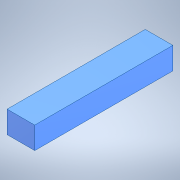
# Autodesk Inventor part: Contenedor Sólido
Saved by Autodesk Inventor 2020.3 (Build 243373000, 373)
## iProperties
Created: 2020-07-19
Part Number: Contenedor Sólido
Material: ABS Plastic
Document SubType Name: Modeling
Designer: juanp
Density: 1.06 g/cm^3
Appearance: Smooth - White
Author: juanp
Autodesk Inventor part; units mm, degrees
ref_plane "YZ Plane" through (0, 0, 0) normal (1, 0, 0) x (0, 1, 0)
ref_plane "XZ Plane" through (0, 0, 0) normal (0, 1, 0) x (-1, 0, 0)
ref_plane "XY Plane" through (0, 0, 0) normal (0, 0, 1) x (1, 0, 0)
sketch "Sketch1" plane through (0, 0, 0) normal (0, 1, 0) x (-1, 0, 0)
  line L0 (0, 0) -> (80, 0)
  line L1 (80, 0) -> (80, -400)
  line L2 (80, -400) -> (0, -400)
  line L3 (0, -400) -> (0, 0)
  line L4 (76, -4) -> (42, -4)
  line L5 (42, -4) -> (42, -39.6)
  line L6 (42, -39.6) -> (76, -39.6)
  line L7 (76, -39.6) -> (76, -4)
  line L8 (76, -43.6) -> (42, -43.6)
  line L9 (42, -43.6) -> (42, -79.2)
  line L10 (42, -79.2) -> (76, -79.2)
  line L11 (76, -79.2) -> (76, -43.6)
  line L12 (76, -83.2) -> (42, -83.2)
  line L13 (42, -83.2) -> (42, -118.8)
  line L14 (42, -118.8) -> (76, -118.8)
  line L15 (76, -118.8) -> (76, -83.2)
  line L16 (76, -122.8) -> (42, -122.8)
  line L17 (42, -122.8) -> (42, -158.4)
  line L18 (42, -158.4) -> (76, -158.4)
  line L19 (76, -158.4) -> (76, -122.8)
  line L20 (76, -162.4) -> (42, -162.4)
  line L21 (42, -162.4) -> (42, -198)
  line L22 (42, -198) -> (76, -198)
  line L23 (76, -198) -> (76, -162.4)
  line L24 (76, -202) -> (42, -202)
  line L25 (42, -202) -> (42, -237.6)
  line L26 (42, -237.6) -> (76, -237.6)
  line L27 (76, -237.6) -> (76, -202)
  line L28 (76, -241.6) -> (42, -241.6)
  line L29 (42, -241.6) -> (42, -277.2)
  line L30 (42, -277.2) -> (76, -277.2)
  line L31 (76, -277.2) -> (76, -241.6)
  line L32 (76, -281.2) -> (42, -281.2)
  line L33 (42, -281.2) -> (42, -316.8)
  line L34 (42, -316.8) -> (76, -316.8)
  line L35 (76, -316.8) -> (76, -281.2)
  line L36 (76, -320.8) -> (42, -320.8)
  line L37 (42, -320.8) -> (42, -356.4)
  line L38 (42, -356.4) -> (76, -356.4)
  line L39 (76, -356.4) -> (76, -320.8)
  line L40 (38, -4) -> (4, -4)
  line L41 (4, -4) -> (4, -39.6)
  line L42 (4, -39.6) -> (38, -39.6)
  line L43 (38, -39.6) -> (38, -4)
  line L44 (38, -43.6) -> (4, -43.6)
  line L45 (4, -43.6) -> (4, -79.2)
  line L46 (4, -79.2) -> (38, -79.2)
  line L47 (38, -79.2) -> (38, -43.6)
  line L48 (38, -83.2) -> (4, -83.2)
  line L49 (4, -83.2) -> (4, -118.8)
  line L50 (4, -118.8) -> (38, -118.8)
  line L51 (38, -118.8) -> (38, -83.2)
  line L52 (38, -122.8) -> (4, -122.8)
  line L53 (4, -122.8) -> (4, -158.4)
  line L54 (4, -158.4) -> (38, -158.4)
  line L55 (38, -158.4) -> (38, -122.8)
  line L56 (38, -162.4) -> (4, -162.4)
  line L57 (4, -162.4) -> (4, -198)
  line L58 (4, -198) -> (38, -198)
  line L59 (38, -198) -> (38, -162.4)
  line L60 (38, -202) -> (4, -202)
  line L61 (4, -202) -> (4, -237.6)
  line L62 (4, -237.6) -> (38, -237.6)
  line L63 (38, -237.6) -> (38, -202)
  line L64 (38, -241.6) -> (4, -241.6)
  line L65 (4, -241.6) -> (4, -277.2)
  line L66 (4, -277.2) -> (38, -277.2)
  line L67 (38, -277.2) -> (38, -241.6)
  line L68 (38, -281.2) -> (4, -281.2)
  line L69 (4, -281.2) -> (4, -316.8)
  line L70 (4, -316.8) -> (38, -316.8)
  line L71 (38, -316.8) -> (38, -281.2)
  line L72 (38, -320.8) -> (4, -320.8)
  line L73 (4, -320.8) -> (4, -356.4)
  line L74 (4, -356.4) -> (38, -356.4)
  line L75 (38, -356.4) -> (38, -320.8)
  line L76 (76, -360.4) -> (4, -360.4)
  line L77 (4, -360.4) -> (4, -396)
  line L78 (4, -396) -> (76, -396)
  line L79 (76, -396) -> (76, -360.4)
  dimension "d0" = 80
  dimension "d1" = 400
  dimension "d2" = 4
  dimension "d3" = 4
  dimension "d4" = 34
  dimension "d5" = 35.6
  dimension "d8" = 39.6
  dimension "d11" = 38
  dimension "d14" = 4
  dimension "d15" = 4
  dimension "d16" = 4
  dimension "d17" = 4
  constraints: 160 end point, 6 parallel, 4 horizontal, 3 perpendicular, 1 vertical, 136 other
  measures "d0" distance of L1.end L2.end
  measures "d1" distance of L0.end L1.end
  measures "d2" distance between parallel lines of L1 L7
  measures "d3" distance between parallel lines of L0 L4
  measures "d4" distance of L5.end L6.end
  measures "d5" distance between parallel lines of L4 L6
  measures "d8" distance of L4.start L8.start
  measures "d11" distance of L4.start L40.start
  measures "d14" distance between parallel lines of L76 L74
  measures "d15" distance between parallel lines of L2 L78
  measures "d16" distance between parallel lines of L3 L77
  measures "d17" distance between parallel lines of L79 L1
extrude "Extrusion1" add sketch "Sketch1" along normal blind 60
sketch "Sketch2" plane through (0, 60, 0) normal (0, 1, 0) x (1, 0, 0)
  line L0 (-80, 0) -> (0, 0) projected
  line L1 (0, 400) -> (-80, 400) projected
  line L2 (-80, 0) -> (0, 0)
  line L3 (0, 0) -> (0, 400)
  line L4 (0, 400) -> (-80, 400)
  line L5 (-80, 400) -> (-80, 0)
  constraints: 8 end point, 2 parallel, 1 horizontal, 1 perpendicular
extrude "Extrusion2" add sketch "Sketch2" along normal blind 4
body "Solid1"
